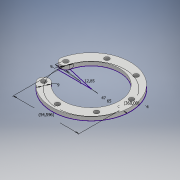
# Autodesk Inventor part: fin entraineur
Saved by Autodesk Inventor 2018.1 (Build 221171000, 171)
## iProperties
Created: 2022-06-22
Part Number: fin entraineur
Material: Generic
Document SubType Name: Modeling
Designer: mouta
Density: 1 g/cm^3
Appearance: Default
Author: mouta
Autodesk Inventor part; units mm, degrees
ref_plane "YZ Plane" through (0, 0, 0) normal (1, 0, 0) x (0, 1, 0)
ref_plane "XZ Plane" through (0, 0, 0) normal (0, 1, 0) x (-1, 0, 0)
ref_plane "XY Plane" through (0, 0, 0) normal (0, 0, 1) x (1, 0, 0)
sketch "Sketch1" plane through (0, 0, 0) normal (0, 0, 1) x (1, 0, 0)
  arc A0 (-25.407, -20.2666) -> (-31.6861, 7.228) centre (0, 0) ccw
  arc A1 (-18.3712, -14.6543) -> (-22.9115, 5.2264) centre (0, 0) ccw
  circle A2 centre (27.2972, 6.234) radius 2
  circle A3 centre (12.1456, 25.2286) radius 2
  circle A4 centre (-12.1519, 25.2256) radius 2
  circle A5 centre (-27.2988, 6.2272) radius 2
  circle A6 centre (-21.8891, -17.4604) radius 2
  circle A7 centre (0.0035, -28) radius 2
  circle A8 centre (21.8935, -17.455) radius 2
  arc A9 (-18.3712, -14.6543) -> (-25.407, -20.2666) centre (-21.8891, -17.4604) ccw
  arc A10 (-31.6861, 7.228) -> (-22.9115, 5.2264) centre (-27.2988, 6.2272) ccw
  line L0 (0, 0) -> (-27.2988, 6.2272)
  line L1 (0, 0) -> (-28.0096, 0)
  dimension "d0" = 65
  dimension "d1" = 47
  dimension "d2" = 4
  dimension "d5" = 360
  dimension "d7" = 9
  dimension "d8" = 9
  dimension "d11" = 12.85
  dimension "d12" = 54.596
  constraints: 11 centre point, 8 point on circle, 4 coincident, 4 end point, 1 horizontal, 15 other
  measures "d0" diameter of A0
  measures "d1" diameter of A1
  measures "d2" diameter of A2
  measures "d7" diameter of A9
  measures "d8" diameter of A10
  measures "d11" angle of L1 L0
  measures "d12" distance of A2.centre A5.centre
extrude "Extrusion1" add sketch "Sketch1" along normal blind 3
body "Solid1"
